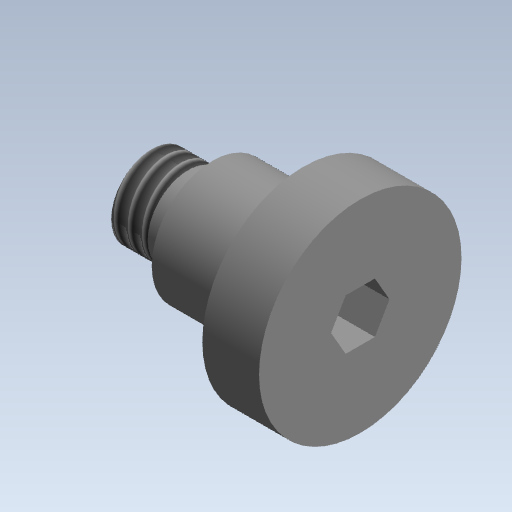
# Autodesk Inventor part: DBTS4-4_5-5-LTC_mod
Saved by Autodesk Inventor 2020.4 (Build 244396000, 396)
## iProperties
Part Number: DBTS4-4_5-5-LTC_mod
Material: 一般
Catalog Web Link: https://jp.misumi-ec.com/vona2/detail/110302679110/?HissuCode=DBTS4-4.5-5-LTC
Description: 既製品
Vendor: MISUMI
Document SubType Name: Modeling
Designer: partserver
Manufacturer: MISUMI
Mass: 0.394189 g
Surface Area: 4.11707 cm^2
Volume: 0.394189 cm^3
Density: 1 g/cm^3
Appearance: PSOLRGB-175-175-175
Category: PARTsolutions
Company: MISUMI
PSOL_IDENT_0: {$CADENAS_DATA\23d-libs\misumi\metric\27_screws_nuts\dbtb.prj},208 {VTYP=3D},{NB=DBTS4-4.5-5-LTC},{L
PSOL_IDENT_1: INA=DBTS4-4.5-5-LTC},{NN=DBTB, DBTM, DBTS},{DATE=03.06.2021 03:35:29},{GEOMDATE=06.03.2020 06:09:28}
PSOL_IDENT_2: ,{VERSION=},{LINEID=20},{WBVAR=MAT,ST,ALT1,L,F,ALT2,ALT3},{WBNUMERIC=L,F}  {NB=DBTS4-4.5-5-LTC},{LIN
PSOL_IDENT_3: A=DBTS4-4.5-5-LTC},{KT=DUMMY},{PN=DBTS4-4.5-5-LTC},{TYPE=DBTS},{MAT=2},{ST=0},{ST0='0','-'},{M=4},{A
PSOL_IDENT_4: LT1=-LTC},{L=4.5},{F=5},{FA=(3:9/1)},{E=2.8},{D=6},{A=10},{B=2.5},{LL=1.2},{HH1=2.5},{P=0.7},{ALT2=}
PSOL_IDENT_5: ,{GG=0.0},{FF=0.0},{LINC=[3:20/0.1] },{ALT3=},{TOL=0/-0.2}
NB: DBTS4-4.5-5-LTC
NN: DBTB, DBTM, DBTS
NT: Stepped Bolts - Low Head Type
NBSYN: $PN.
LINA: DBTS4-4.5-5-LTC
CATALOG: Misumi
PN: DBTS4-4.5-5-LTC
MAT: 303 Stainless Steel
ST: -
M: 4
ALT1: with LTC (L Dimension Increment)
L: 4.5
F: 5
E: 2.8
D: 6
A: 10
B: 2.5
LL: 1.2
HH1: 2.5
ALT2: w/o PC (Relief on M)
ALT3: w/o DHC (Shaft Diameter Tolerance)
TOL: 0/-0.2
SUPPLIER: MISUMI
ARTICLENO: DBTS4-4.5-5-LTC
BOMINFO: DBTS4-4.5-5-LTC
CREATOR: CADENAS GmbH
Title: DBTS4-4.5-5-LTC
Author: Cadenas PARTsolutions
Comments: Stepped Bolts - Low Head Type
Autodesk Inventor part; units mm, degrees
ref_plane "YZ Plane" through (0, 0, 0) normal (1, 0, 0) x (0, 1, 0)
ref_plane "XZ Plane" through (0, 0, 0) normal (0, 1, 0) x (-1, 0, 0)
ref_plane "XY Plane" through (0, 0, 0) normal (0, 0, 1) x (1, 0, 0)
sketch "Sketch_1" plane through (0, 0, 0) normal (0, 0, 1) x (1, 0, 0)
  line L0 (4.5, 0) -> (-2.8, 0)
  line L1 (-2.8, 0) -> (-2.8, 5)
  line L2 (-2.8, 5) -> (0, 5)
  line L3 (0, 5) -> (0, 3)
  line L4 (0, 3) -> (4.5, 3)
  line L5 (4.5, 3) -> (4.5, 0)
  line L6 (4.5, 0) -> (-2.8, 0)
  constraints: 14 end point
revolve "Revolution1" add sketch "Sketch_1" angle 360 about axis through (4.5, 0, 0) along (1, 0, 0)
sketch "Sketch2" plane through (-2.8, 0, 0) normal (-1, 0, 0) x (0, 0, 1)
  point P0 (0, 0)
hole "Hole1" at (-2.8, 0, 0) direction (1, 0, 0) diameter 2.5 depth 2.5 tip angle 120
sketch "Sketch_3" plane through (-2.8, 0, 0) normal (1, 0, 0) x (0, 0, -1)
  line L0 (-1.25, -0.7217) -> (0, -1.4434)
  line L1 (0, -1.4434) -> (1.25, -0.7217)
  line L2 (1.25, -0.7217) -> (1.25, 0.7217)
  line L3 (1.25, 0.7217) -> (0, 1.4434)
  line L4 (0, 1.4434) -> (-1.25, 0.7217)
  line L5 (-1.25, 0.7217) -> (-1.25, -0.7217)
  constraints: 12 end point
extrude "Extrusion1" cut sketch "Sketch_3" along normal blind 2.5
sketch "Sketch_6" plane through (0, 0, 0) normal (0, 0, 1) x (1, 0, 0)
  line L0 (9.5, 0) -> (4.5, 0)
  line L1 (4.5, 0) -> (4.5, 2)
  line L2 (4.5, 2) -> (9.0705, 2)
  line L3 (9.0705, 2) -> (9.5, 1.5705)
  line L4 (9.5, 1.5705) -> (9.5, 0)
  line L5 (9.5, 0) -> (4.5, 0)
  constraints: 12 end point
revolve "Revolution2" add sketch "Sketch_6" angle 360 about axis through (9.5, 0, 0) along (1, 0, 0)
thread "Thread1" size "M4x0.7" class "6g" standard "ISO Metric profile" length 3.3705
sketch "スケッチ5" plane through (9.5, 0, 0) normal (1, 0, 0) x (0, 0, -1)
  circle A0 centre (0, 0) radius 5
  constraints: 1 centre point, 1 coincident
extrude "押し出し2" cut sketch "スケッチ5" against normal blind 2
body "Solid1"
